Autodesk Fusion 360 part; units mm, degrees
(part 2 of 2)
  line L451 (111, -240) -> (120, -240)
  line L452 (120, -210) -> (120, -219)
  line L453 (120, -219) -> (111, -219)
  line L454 (111, -219) -> (111, -210)
  line L455 (111, -210) -> (120, -210)
  line L456 (120, -220) -> (120, -229)
  line L457 (120, -229) -> (111, -229)
  line L458 (111, -229) -> (111, -220)
  line L459 (111, -220) -> (120, -220)
  line L460 (110, -90) -> (110, -99)
  line L461 (110, -99) -> (101, -99)
  line L462 (101, -99) -> (101, -90)
  line L463 (101, -90) -> (110, -90)
  line L464 (120, -230) -> (120, -239)
  line L465 (120, -239) -> (111, -239)
  line L466 (111, -239) -> (111, -230)
  line L467 (111, -230) -> (120, -230)
  line L468 (120, -200) -> (120, -209)
  line L469 (120, -209) -> (111, -209)
  line L470 (111, -209) -> (111, -200)
  line L471 (111, -200) -> (120, -200)
  line L472 (120, -190) -> (120, -199)
  line L473 (120, -199) -> (111, -199)
  line L474 (111, -199) -> (111, -190)
  line L475 (111, -190) -> (120, -190)
  line L476 (120, -180) -> (120, -189)
  line L477 (120, -189) -> (111, -189)
  line L478 (111, -189) -> (111, -180)
  line L479 (111, -180) -> (120, -180)
  line L480 (120, -170) -> (120, -179)
  line L481 (120, -179) -> (111, -179)
  line L482 (111, -179) -> (111, -170)
  line L483 (111, -170) -> (120, -170)
  line L484 (120, -160) -> (120, -169)
  line L485 (120, -169) -> (111, -169)
  line L486 (111, -169) -> (111, -160)
  line L487 (111, -160) -> (120, -160)
  line L488 (120, -150) -> (120, -159)
  line L489 (120, -159) -> (111, -159)
  line L490 (111, -159) -> (111, -150)
  line L491 (111, -150) -> (120, -150)
  line L492 (120, -140) -> (120, -149)
  line L493 (120, -149) -> (111, -149)
  line L494 (111, -149) -> (111, -140)
  line L495 (111, -140) -> (120, -140)
  line L496 (120, -130) -> (120, -139)
  line L497 (120, -139) -> (111, -139)
  line L498 (111, -139) -> (111, -130)
  line L499 (111, -130) -> (120, -130)
  line L500 (120, -120) -> (120, -129)
  line L501 (120, -129) -> (111, -129)
  line L502 (111, -129) -> (111, -120)
  line L503 (111, -120) -> (120, -120)
  line L504 (120, -110) -> (120, -119)
  line L505 (120, -119) -> (111, -119)
  line L506 (111, -119) -> (111, -110)
  line L507 (111, -110) -> (120, -110)
  line L508 (111, -90) -> (120, -90)
  line L509 (120, -90) -> (120, -99)
  line L510 (120, -99) -> (111, -99)
  line L511 (111, -99) -> (111, -90)
  line L512 (40, -250) -> (121, -250)
  line L513 (121, -250) -> (121, -89)
  line L514 (121, -89) -> (40, -89)
  line L515 (40, -89) -> (40, -250)
  line L516 (40, -89) -> (35, -89)
  line L517 (35, -89) -> (35, -84)
  line L518 (121, -250) -> (126, -250)
  line L519 (126, -250) -> (126, -255)
  line L520 (126, -255) -> (35, -255)
  line L521 (35, -255) -> (35, -84)
  line L522 (35, -84) -> (126, -84)
  line L523 (126, -84) -> (126, -255)
  constraint coincident L514.end L515.start
  constraint perpendicular L515 L516
  constraint perpendicular L516 L517
  constraint coincident L512.end L513.start
  constraint perpendicular L513 L518
  constraint perpendicular L512 L519
  constraint horizontal L520
  constraint vertical L521
  constraint horizontal L522
  constraint vertical L523
extrude "Extruir13" add sketch "Boceto14" against normal blind 2 contours L512 L515 L516 L518 L519 L520 L521 L523 | L513 L514 L516 L517 L518 L521 L522 L523 bodies 1
extrude "Extruir14" cut 1 faces at (120.6667, 153, 10) along direction (0, 0, -1) blind 2 on bodies 1 bodies 1
fillet "Empalme1" radius 3 4 edges at (126, 255, 1) (35, 255, 1) (126, 84, 1) (35, 84, 1) on bodies 1
